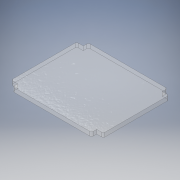
# Autodesk Inventor part: BT701_trajan20_21
Saved by Autodesk Inventor 2022.2 (Build 262287000, 287)
## iProperties
Company: HTBLA Kaindorf
RuleStatus: InUse
Created: 2022-08-21
Part Number: BT701_trajan20_21
Project: Zeichenmaschine_v2
Material: Acryl
Description: Plexi_100x80
Document SubType Name: Modeling
Designer: trajan20
Density: 1.188 g/cm^3
Appearance: Transparent - farblos
Mass: 60.6817 g
Surface Area: 224.492 cm^2
Volume: 51.0789 cm^3
AfterDocNew0: iProperties-Editor_aufrufen
Author: jan
Keywords: 2021
Autodesk Inventor part; units mm, degrees
ref_plane "YZ Plane" through (0, 0, 0) normal (1, 0, 0) x (0, 1, 0)
ref_plane "XZ Plane" through (0, 0, 0) normal (0, 1, 0) x (-1, 0, 0)
ref_plane "XY Plane" through (0, 0, 0) normal (0, 0, 1) x (1, 0, 0)
sketch "Skizze3" plane through (0, 0, 0) normal (0, 0, 1) x (1, 0, 0)
  line L0 (0, 0) -> (-80, 0)
  line L1 (-80, 0) -> (-80, 100)
  line L2 (-80, 100) -> (0, 100)
  line L3 (0, 100) -> (0, 0)
  line L4 (-80, 100) -> (0, 100)
  line L5 (-40, 106.3) -> (-80, 106.3)
  line L6 (-80, 106.3) -> (-80, 100)
  line L7 (-80, 50) -> (-86.3, 50)
  line L8 (-86.3, 50) -> (-86.3, 98.2)
  line L9 (-86.3, 98.2) -> (-80, 98.2)
  line L10 (-80, 98.2) -> (-80, 50)
  line L11 (-40, 106.3) -> (-40, 100)
  dimension "d4" = 100
  dimension "d5" = 80
  dimension "d6" = 6.3
  dimension "d7" = 6.3
  dimension "d8" = 1.8
  constraints: 24 end point, 5 parallel, 4 midpoint, 3 horizontal, 3 perpendicular, 2 point on line
  measures "d4" distance between parallel lines of L2 L0
  measures "d5" distance between parallel lines of L1 L3
  measures "d6" distance between parallel lines of L2 L5
  measures "d7" distance between parallel lines of L8 L1
  measures "d8" distance between parallel lines of L2 L9
extrude "Extrusion3" add sketch "Skizze3" along normal blind 5 contours L0 L1 L2 L3
extrude "Extrusion4" add sketch "Skizze3" along normal blind 5 contours L7 L8 L9 L1 | L2 L6 L5 L11
fillet "Rundung1" radius 2 2 edges at (-86.3, 98.2, 2.5) (-80, 106.3, 2.5)
mirror "Spiegeln1" about plane through (-86.3, 50, 0) normal (0, -1, 0) of "Extrusion4", "Rundung1"
mirror "Spiegeln2" about plane through (-40, 0, 0) normal (1, 0, 0) of "Extrusion4", "Rundung1", "Spiegeln1"
equation "\"d7\" = d6"
